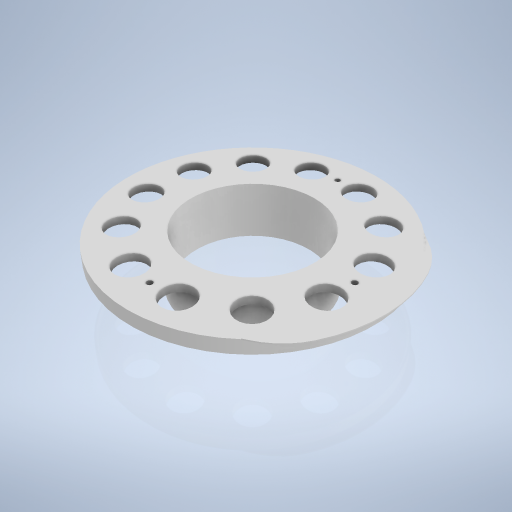
# Autodesk Inventor part: nockenscheibe
Saved by Autodesk Inventor 2024.2 (Build 282272000, 272)
## iProperties
Created: 2024-04-30
Part Number: nockenscheibe
Material: Generisch
Document SubType Name: Modeling
Designer: ffogue
Density: 1 g/cm^3
Appearance: Vorgabe
Author: ffogue
Autodesk Inventor part; units mm, degrees
note: some values were not read from the file. Chosen so that the rebuilt part matches the saved one: direction of "Bohrung1"; direction of "Bohrung2".
ref_plane "YZ Plane" through (0, 0, 0) normal (1, 0, 0) x (0, 1, 0)
ref_plane "XZ Plane" through (0, 0, 0) normal (0, 1, 0) x (-1, 0, 0)
ref_plane "XY Plane" through (0, 0, 0) normal (0, 0, 1) x (1, 0, 0)
sketch "Skizze1" plane through (0, 0, 0) normal (0, 1, 0) x (-1, 0, 0)
  line L0 (17.5, 0) -> (35, 0)
  line L1 (35, 0) -> (35, -0.3)
  line L2 (35, -0.3) -> (35, -0.3)
  line L3 (35, -0.3) -> (35, -3.5)
  line L4 (19, -3.5) -> (19, -14)
  line L5 (19, -14) -> (17.5, -14)
  line L6 (17.5, -14) -> (17.5, 0)
  line L7 (0, 0) -> (0, -14)
  line L8 (35, -3.5) -> (35, -3.5)
  line L9 (33, -2) -> (20.5, -2)
  line L10 (20.5, -2) -> (20.5, -2)
  line L11 (35, -3.5) -> (35, -3.5)
  line L12 (20.5, -2) -> (20.5, -2)
  arc A0 (20.5, -2) -> (19, -3.5) centre (20.5, -3.5) ccw
  line L13 (34.5, -3.5) -> (34.5, -3.5)
  line L14 (34.5, -3.5) -> (35, -3.5)
  arc A1 (34.5, -3.5) -> (33, -2) centre (33, -3.5) ccw
  point P0 (19, -2)
  point P1 (35, -2)
  point P2 (34.5, -2)
  point P3 (0, -7)
  dimension "d1" = 14
  dimension "d3" = 35
  dimension "d4" = 38
  dimension "d5" = 70
  dimension "d10" = 2
  dimension "d11" = 1.5
  dimension "d34" = 69
  dimension "d35" = 1.5
  dimension "d36" = 3.5
  constraints: 30 end point, 13 perpendicular, 6 point on line, 4 point on circle, 4 tangent, 3 horizontal alignment, 2 centre point, 2 horizontal, 2 vertical, 2 vertical alignment, 1 collinear, 1 midpoint, 1 parallel
  measures "d1" distance of L7.start L7.end
  measures "d3" diameter of L6 L7
  measures "d4" diameter of L4 L7
  measures "d5" diameter of L3 L7
  measures "d10" distance between parallel lines of L9 L0
  measures "d11" radius of A0
  measures "d34" diameter of L13 point (0, -7)
  measures "d35" radius of A1
  measures "d36" distance from line of L0 A1.centre
revolve "Umdrehung1" add sketch "Skizze1" angle 360 about axis through (0, 0, 0) along (0, 0, -1)
sketch "Skizze2" plane through (0, 0, 0) normal (0, 0, 1) x (1, 0, 0)
  line L0 (0, 0) -> (0, 36.826) construction
  circle A0 centre (0, 0) radius 27 construction
  line L1 (0, 0) -> (-10.2306, 38.1811) construction
  line L2 (0, 0) -> (20.6417, 35.7525) construction
  point P0 (-6.9881, 26.08)
  dimension "d13" = 54
  dimension "d14" = 30
  dimension "d15" = 45
  constraints: 6 end point, 1 coincident, 1 point on line, 1 vertical, 3 other
  measures "d14" angle of L0 L2
  measures "d15" angle of L1 L2
hole "Bohrung1" at (-6.9881, 26.08, 0) direction (0, 0, -1) diameter 8 depth 2
pattern_circular "Runde Anordnung1" count 12 over 360 about axis through (0, 0, -7) along (0, 0, -1) of "Bohrung1"
sketch "Skizze3" plane through (0, 0, 0) normal (0, 0, 1) x (1, 0, 0)
  circle A0 centre (0, 0) radius 27 construction
  point P0 (0, 0)
  point P1 (0, 27)
  point P2 (0, -27)
  point P3 (27, 0)
  dimension "d33" = 54
  constraints: 3 point on circle, 1 centre point, 1 coincident, 1 vertical alignment
  measures "d33" diameter of A0
hole "Bohrung2" at (0, 27, 0) at (0, -27, 0) at (27, 0, 0) direction (0, 0, -1) diameter 1.567 depth 2 thread size "M2x0.4" class "6H" standard "ISO Metric profile"
sketch "Skizze4" plane through (0, 0, 0) normal (0, 0, 1) x (1, 0, 0)
  circle A0 centre (0, 0) radius 35 projected
  line L0 (0, 0) -> (68.1338, 0) construction
  arc A1 (32.619, -17.4643) -> (34.9596, 12.1171) centre (0, 0) ccw
  arc A2 (34.9596, 12.1171) -> (28.6608, 20.9014) centre (17.0074, 5.8948) ccw
  circle A3 centre (0, 0) radius 35 projected
  arc A4 (25.4755, 24) -> (28.6608, 20.9014) centre (40.9275, 36.6979) ccw
  arc A5 (24.44, -25.4529) -> (32.619, -17.4643) centre (15.8687, -8.4961) ccw
  arc A6 (24.44, -25.4529) -> (23.4307, -26) centre (33.4625, -43.3021) ccw
  point P0 (0, 0)
  point P1 (25.5164, 23.9565)
  point P2 (26.6259, 22.717)
  dimension "d43" = 74
  dimension "d47" = 19
  dimension "d48" = 20
  dimension "d49" = 19
  dimension "d50" = 20
  dimension "d51" = 50
  dimension "d52" = 80
  dimension "d53" = 24
  dimension "d54" = 26
  constraints: 13 point on circle, 5 centre point, 4 tangent, 2 end point, 1 coincident, 1 horizontal
  measures "d43" diameter of A1
  measures "d47" radius of A2
  measures "d48" radius of A4
  measures "d49" radius of A5
  measures "d50" radius of A6
  measures "d51" distance of A0.start A0.end
  measures "d52" vertical distance of A6.centre A4.centre
  measures "d53" distance from line of L0 A4.start
  measures "d54" distance from line of L0 A0.start
extrude "Extrusion1" add sketch "Skizze4" along normal mid plane 0.3 contours A0 A4 A2 A1 A5 A6
